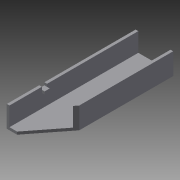
# Autodesk Inventor part: Horizontal channel
Saved by Autodesk Inventor 2014 SP1 (Build 180222100, 222)
## iProperties
Created: 2015-02-04
Part Number: Horizontal channel
Material: Generic
Document SubType Name: Modeling
Designer: degan
Density: 1 g/cm^3
Appearance: Default
Author: degan
Autodesk Inventor part; units mm, degrees
ref_plane "YZ Plane" through (0, 0, 0) normal (1, 0, 0) x (0, 1, 0)
ref_plane "XZ Plane" through (0, 0, 0) normal (0, 1, 0) x (-1, 0, 0)
ref_plane "XY Plane" through (0, 0, 0) normal (0, 0, 1) x (1, 0, 0)
sketch "Sketch1" plane through (0, 0, 0) normal (0, 0, 1) x (1, 0, 0)
  line L0 (24.1101, 25.4) -> (24.1101, 0)
  line L1 (24.1101, 0) -> (-20.3399, 0)
  line L2 (-20.3399, 0) -> (-20.3399, 25.4)
  line L3 (-17.1649, 25.4) -> (-17.1649, 3.175)
  line L4 (-17.1649, 3.175) -> (20.9351, 3.175)
  line L5 (20.9351, 3.175) -> (20.9351, 25.4)
  line L6 (-20.3399, 25.4) -> (-17.1649, 25.4)
  line L7 (24.1101, 25.4) -> (20.9351, 25.4)
  point P0 (0, 0)
  dimension "d0" = 44.45
  dimension "d1" = 25.4
  dimension "d2" = 3.175
  constraints: 16 end point, 3 equal length, 1 perpendicular, 2 other
  measures "d0" distance of L0.end L1.end
  measures "d1" distance of L1.end L2.end
  measures "d2" distance between parallel lines of L0 L5
extrude "Extrusion1" add sketch "Sketch1" against normal blind 152.4
sketch "Sketch3" plane through (-20.3399, 0, 0) normal (-1, 0, 0) x (0, 0, 1)
  line L0 (0, 25.4) -> (-152.4, 25.4) projected
  line L1 (-152.4, 0) -> (-152.4, 25.4) projected
  line L2 (0, 0) -> (-152.4, 0) projected
  line L3 (-44.45, 25.4) -> (-44.45, 19.05)
  line L4 (-44.45, 19.05) -> (-38.354, 19.05)
  line L5 (-38.354, 19.05) -> (-38.354, 25.4)
  dimension "d6" = 6.096
  dimension "d7" = 6.35
  dimension "d8" = 107.95
  constraints: 6 end point, 3 perpendicular, 2 point on line
  measures "d6" distance of L5.end L3.start
  measures "d7" distance of L3.start L3.end
  measures "d8" distance between parallel lines of L1 L3
extrude "Extrusion2" cut sketch "Sketch3" against normal up to next
sketch "Sketch4" plane through (-20.3399, 0, 0) normal (-1, 0, 0) x (0, 0, 1)
  line L0 (-38.354, 19.05) -> (-44.45, 19.05) projected
  line L1 (-44.45, 19.05) -> (-44.45, 22.225)
  line L2 (-44.45, 25.4) -> (-44.45, 19.05) projected
  line L3 (-38.354, 19.05) -> (-38.354, 25.4) projected
  line L4 (-38.354, 19.05) -> (-44.45, 19.05)
  line L5 (-44.45, 19.05) -> (-38.354, 19.05) projected
  line L6 (-44.45, 22.225) -> (-38.354, 22.225)
  line L7 (-38.354, 19.05) -> (-38.354, 22.225)
  dimension "d11" = 3.175
  constraints: 8 end point, 2 midpoint, 1 collinear
  measures "d11" distance of L0.end L1.end
extrude "Extrusion3" add sketch "Sketch4" against normal blind 6.35
sketch "Sketch5" plane through (-20.3399, 0, 0) normal (0, -1, 0) x (1, 0, 0)
  line L0 (0, 0) -> (44.45, 0) projected
  line L1 (44.45, 0) -> (44.45, -152.4) projected
  line L2 (44.45, -152.4) -> (44.45, -41.275)
  line L3 (44.45, 0) -> (44.45, -152.4) projected
  line L4 (44.45, -41.275) -> (12.2024, 0)
  line L5 (12.2024, 0) -> (44.45, 0)
  line L6 (44.45, 0) -> (44.45, -41.275)
  point P0 (20.3399, 0)
  dimension "d14" = 111.125
  dimension "d15" = 38
  constraints: 8 end point, 2 point on line, 1 collinear, 1 perpendicular
  measures "d14" distance of L1.end L2.end
  measures "d15" angle of L4 L1
extrude "Extrusion4" cut sketch "Sketch5" against normal through all
body "Solid1"
